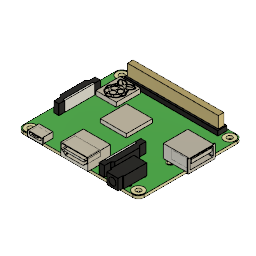
Raspberry PI 3 Model A+ - TG v7 (Autodesk Fusion 360 design; units mm, degrees)
Autodesk Fusion 360 part; units mm, degrees
note: some values were not read from the file. Set by a fixed rule: which sketch regions a step uses.
(part 1 of 2)
sketch "Board Outline" plane through (0, 0, 0) normal (0, 0, 1) x (1, 0, 0)
  arc A0 (0, 3) -> (3, 0) centre (3, 3) ccw
  line L0 (3, 0) -> (62, 0)
  line L1 (0, 53) -> (0, 3)
  arc A1 (3, 56) -> (0, 53) centre (3, 53) ccw
  circle A2 centre (61.5, 52.5) radius 3
  circle A3 centre (3.5, 52.5) radius 1.4
  arc A4 (65, 53) -> (62, 56) centre (62, 53) ccw
  circle A5 centre (61.5, 3.5) radius 1.4
  circle A6 centre (3.5, 3.5) radius 1.4
  arc A7 (62, 0) -> (65, 3) centre (62, 3) ccw
  circle A8 centre (61.5, 52.5) radius 1.4
  circle A9 centre (3.5, 52.5) radius 3
  circle A10 centre (61.5, 3.5) radius 3
  line L2 (65, 3) -> (65, 53)
  line L3 (62, 56) -> (3, 56)
  circle A11 centre (3.5, 3.5) radius 3
extrude "Extrude1" add sketch "Board Outline" along normal blind 1.5 contours A0 L0 L1 A1 A4 A7 L2 L3 makes body 1
extrude "Extrude2" add sketch "Board Outline" along normal blind 1.49 contours A2 | A9 | A10 | A11 bodies 1
sketch "Bottom Mounting Pads" plane through (0, 0, 0) normal (0, 0, -1) x (1, 0, 0)
  circle A0 centre (61.5, -3.5) radius 1.4
  circle A1 centre (3.5, -3.5) radius 1.4
  circle A2 centre (61.5, -52.5) radius 1.4
  circle A3 centre (3.5, -52.5) radius 1.4
  line L0 (3, -56) -> (62, -56)
  arc A4 (62, -56) -> (65, -53) centre (62, -53) ccw
  line L1 (65, -53) -> (65, -3)
  arc A5 (65, -3) -> (62, 0) centre (62, -3) ccw
  line L2 (62, 0) -> (3, 0)
  arc A6 (3, 0) -> (0, -3) centre (3, -3) ccw
  line L3 (0, -3) -> (0, -53)
  arc A7 (0, -53) -> (3, -56) centre (3, -53) ccw
extrude "Extrude3" cut sketch "Board Outline" along normal blind 0.01 contours A2 | A9 | A10 | A11 bodies 1
sketch "Components - Top" plane through (0, 0, 1.5) normal (0, 0, 1) x (1, 0, 0)
  line L0 (46.35, 19.35) -> (46.35, 22.7)
  line L1 (46.35, 22.7) -> (43.55, 22.7)
  line L2 (43.55, 22.7) -> (43.55, 0.3)
  line L3 (43.55, 3.5) -> (44.45, 3.5)
  line L4 (47.5, 4.8) -> (47.5, 18.2)
  line L5 (44.45, 19.5) -> (43.55, 19.5)
  line L6 (44.45, 3.5) -> (44.45, 19.5)
  line L7 (6.58, -1.22) -> (14.62, -1.22)
  line L8 (19.975, 24.525) -> (33.975, 24.525)
  line L9 (14.62, -1.22) -> (14.62, -0.6)
  line L10 (39.25, -1.5) -> (39.25, 10.65)
  line L11 (19.975, 38.525) -> (19.975, 24.525)
  line L12 (33.975, 38.525) -> (19.975, 38.525)
  line L13 (14.35, -0.6) -> (14.35, 4.71)
  line L14 (33.975, 24.525) -> (33.975, 38.525)
  line L15 (14.62, -0.6) -> (6.58, -0.6)
  line L16 (24.75, -1.5) -> (39.25, -1.5)
  line L17 (6.58, -0.6) -> (6.58, -1.22)
  line L18 (24.75, 10.65) -> (24.75, -1.5)
  line L19 (6.85, -0.6) -> (14.35, -0.6)
  line L20 (6.85, 4.71) -> (6.85, -0.6)
  line L21 (14.35, 4.71) -> (6.85, 4.71)
  line L22 (2.6, 39.2) -> (2.6, 35.8)
  line L23 (1.5, 21.3) -> (2.65, 20.15)
  line L24 (39.25, 10.65) -> (24.75, 10.65)
  line L25 (2.65, 20.15) -> (2.65, 16.8)
  line L26 (2.65, 16.8) -> (5.45, 16.8)
  line L27 (4.55, 20) -> (5.45, 20)
  line L28 (5.45, 16.8) -> (5.45, 39.2)
  line L29 (5.45, 36) -> (4.55, 36)
  line L30 (1.5, 34.7) -> (1.5, 21.3)
  line L31 (2.6, 35.8) -> (1.5, 34.7)
  line L32 (4.55, 36) -> (4.55, 20)
  line L33 (47.5, 18.2) -> (46.35, 19.35)
  line L34 (5.45, 39.2) -> (2.6, 39.2)
  line L35 (43.55, 0.3) -> (46.4, 0.3)
  line L36 (46.4, 0.3) -> (46.4, 3.7)
  line L37 (46.4, 3.7) -> (47.5, 4.8)
extrude "Extrude4" add sketch "Components - Top" along normal blind 2 separate body contours L8 L11 L12 L14 makes body 2
extrude "Extrude5" add sketch "Components - Top" along normal blind 5.5 separate body contours L0 L1 L2 L3 L4 L5 L6 L33 L35 L36 L37 | L22 L23 L25 L26 L27 L28 L29 L30 L31 L32 L34 makes body 3 at (4.55, 30.6667, 3.3333) makes body 4 at (44.45, 8.8333, 3.3333)
extrude "Extrude6" add sketch "Components - Top" along normal blind 5.51 separate body contours L2 L3 L5 L6 | L27 L28 L29 L32 makes body 5 at (5.45, 25.3333, 3.3367) makes body 6 at (44.45, 8.8333, 3.3367)
extrude "Extrude7" add sketch "Components - Top" along normal blind 6.5 separate body contours L10 L16 L18 L24 makes body 7
extrude "Extrude8" add sketch "Components - Top" along normal blind 3 separate body contours L7 L9 L15 L17 L19 | L13 L15 L19 L20 L21 makes body 8
sketch "Components - Bottom" plane through (0, 0, 0) normal (0, 0, -1) x (-1, 0, 0)
  line L0 (-13.135, 34.1) -> (-13.135, 22.11)
  line L1 (-1.685, 34.1) -> (-13.135, 34.1)
  line L2 (-13.135, 22.11) -> (-1.685, 22.11)
  line L3 (-1.685, 22.11) -> (-1.685, 34.1)
  line L4 (-1.685, 22.51) -> (2.265, 22.51)
  line L5 (-49.6, 39.5) -> (-37.6, 39.5)
  line L6 (2.265, 22.51) -> (2.265, 33.51)
  line L7 (2.265, 33.51) -> (-1.685, 33.51)
  line L8 (-37.6, 39.5) -> (-37.6, 27.5)
  line L9 (-37.6, 27.5) -> (-49.6, 27.5)
  line L10 (-49.6, 27.5) -> (-49.6, 39.5)
extrude "Extrude9" add sketch "Components - Bottom" along normal blind 0.65 separate body contours L5 L8 L9 L10 makes body 9
extrude "Extrude10" add sketch "Components - Bottom" along normal blind 1.45 separate body contours L0 L1 L2 L3 | L3 L4 L6 L7 makes body 10
sketch "Pads" plane through (0, 0, 1.5) normal (0, 0, 1) x (1, 0, 0)
  circle A0 centre (54.5, 30.45) radius 0.75
  circle A1 centre (56.63, 51.23) radius 0.8
  circle A2 centre (57.21, 24.88) radius 1.725
  circle A3 centre (8.37, 53.77) radius 0.8
  circle A4 centre (54.5, 27.95) radius 0.75
  circle A5 centre (50.3, 3.5) radius 0.9
  circle A6 centre (54.5, 32.45) radius 0.75
  circle A7 centre (54.5, 34.95) radius 0.75
  line L0 (9.17, 52.03) -> (9.17, 50.43)
  circle A8 centre (41.39, 51.23) radius 0.8
  circle A9 centre (41.39, 53.77) radius 0.8
  line L1 (7.57, 52.03) -> (9.17, 52.03)
  line L2 (7.57, 50.43) -> (7.57, 52.03)
  circle A10 centre (57.21, 38.02) radius 1.725
  line L3 (9.17, 50.43) -> (7.57, 50.43)
  circle A11 centre (46.47, 51.23) radius 0.8
  circle A12 centre (28.69, 53.77) radius 0.8
  circle A13 centre (38.85, 53.77) radius 0.8
  circle A14 centre (15.99, 51.23) radius 0.8
  circle A15 centre (54.09, 53.77) radius 0.8
  circle A16 centre (49.01, 51.23) radius 0.8
  circle A17 centre (13.45, 53.77) radius 0.8
  circle A18 centre (46.47, 53.77) radius 0.8
  circle A19 centre (21.07, 51.23) radius 0.8
  circle A20 centre (23.61, 51.23) radius 0.8
  circle A21 centre (36.31, 51.23) radius 0.8
  circle A22 centre (10.91, 53.77) radius 0.8
  circle A23 centre (43.93, 51.23) radius 0.8
  circle A24 centre (43.93, 53.77) radius 0.8
  circle A25 centre (21.07, 53.77) radius 0.8
  circle A26 centre (56.63, 53.77) radius 0.8
  circle A27 centre (13.45, 51.23) radius 0.8
  circle A28 centre (26.15, 53.77) radius 0.8
  circle A29 centre (50.6, 11.5) radius 0.475
  circle A30 centre (41.39, 53.77) radius 0.475
  circle A31 centre (36.31, 51.23) radius 0.475
  circle A32 centre (10.91, 51.23) radius 0.8
  circle A33 centre (23.61, 51.23) radius 0.475
  circle A34 centre (49.01, 53.77) radius 0.475
  circle A35 centre (49.01, 51.23) radius 0.475
  circle A36 centre (54.09, 51.23) radius 0.475
  circle A37 centre (28.69, 51.23) radius 0.8
  circle A38 centre (54.5, 34.95) radius 0.475
  circle A39 centre (43.93, 53.77) radius 0.475
  circle A40 centre (51.55, 51.23) radius 0.475
  circle A41 centre (23.61, 53.77) radius 0.8
  circle A42 centre (53.5, 12.2) radius 0.475
  circle A43 centre (56.63, 53.77) radius 0.475
  circle A44 centre (36.31, 53.77) radius 0.475
  circle A45 centre (46.47, 51.23) radius 0.475
  circle A46 centre (54.09, 53.77) radius 0.475
  circle A47 centre (38.85, 51.23) radius 0.475
  circle A48 centre (49.01, 53.77) radius 0.8
  circle A49 centre (54.5, 32.45) radius 0.475
  circle A50 centre (31.23, 53.77) radius 0.475
  circle A51 centre (18.53, 53.77) radius 0.8
  circle A52 centre (33.77, 51.23) radius 0.475
  circle A53 centre (15.99, 53.77) radius 0.8
  circle A54 centre (31.23, 51.23) radius 0.8
  circle A55 centre (54.09, 51.23) radius 0.8
  circle A56 centre (23.61, 53.77) radius 0.475
  circle A57 centre (50.3, 3.5) radius 0.475
  circle A58 centre (18.53, 51.23) radius 0.8
  circle A59 centre (31.23, 53.77) radius 0.8
  circle A60 centre (54.5, 27.95) radius 0.475
  circle A61 centre (53.5, 12.2) radius 0.9
  circle A62 centre (26.15, 53.77) radius 0.475
  circle A63 centre (51.55, 51.23) radius 0.8
  circle A64 centre (56.63, 51.23) radius 0.475
  circle A65 centre (46.47, 53.77) radius 0.475
  circle A66 centre (36.31, 53.77) radius 0.8
  circle A67 centre (33.77, 53.77) radius 0.8
  circle A68 centre (56.7, 3.5) radius 0.475
  circle A69 centre (56.7, 3.5) radius 0.9
  circle A70 centre (41.39, 51.23) radius 0.475
  circle A71 centre (57.21, 38.02) radius 1.15
  circle A72 centre (38.85, 53.77) radius 0.475
  circle A73 centre (57.21, 24.88) radius 1.15
  circle A74 centre (31.23, 51.23) radius 0.475
  circle A75 centre (56.4, 11.5) radius 0.475
  circle A76 centre (51.55, 53.77) radius 0.475
  circle A77 centre (38.85, 51.23) radius 0.8
  circle A78 centre (26.15, 51.23) radius 0.8
  circle A79 centre (43.93, 51.23) radius 0.475
  circle A80 centre (51.55, 53.77) radius 0.8
  circle A81 centre (33.77, 51.23) radius 0.8
  circle A82 centre (56.4, 11.5) radius 0.9
  circle A83 centre (54.5, 30.45) radius 0.475
  circle A84 centre (28.69, 53.77) radius 0.475
  circle A85 centre (50.6, 11.5) radius 0.9
  circle A86 centre (33.77, 53.77) radius 0.475
  circle A87 centre (8.37, 53.77) radius 0.475
  circle A88 centre (15.99, 53.77) radius 0.475
  circle A89 centre (13.45, 51.23) radius 0.475
  circle A90 centre (10.91, 53.77) radius 0.475
  circle A91 centre (10.91, 51.23) radius 0.475
  circle A92 centre (15.99, 51.23) radius 0.475
  circle A93 centre (21.07, 53.77) radius 0.475
  circle A94 centre (28.69, 51.23) radius 0.475
  circle A95 centre (21.07, 51.23) radius 0.475
  circle A96 centre (8.37, 51.23) radius 0.475
  circle A97 centre (13.45, 53.77) radius 0.475
  circle A98 centre (18.53, 53.77) radius 0.475
  circle A99 centre (18.53, 51.23) radius 0.475
  circle A100 centre (26.15, 51.23) radius 0.475
extrude "Extrude11" cut sketch "Pads" against normal blind 0.01 contours L0 L1 L2 L3 bodies 1
hole "Hole2" at (56.63, 53.77, 1.5) direction (0, 0, -1) diameter 0.95 depth 1.5 tip angle 118 counterbore diameter 1.6 counterbore depth 0.01 bodies 1
sketch "Sketch14" plane through (0, 0, 0) normal (0, 0, -1) x (1, 0, 0)
  line L0 (3, -56) -> (62, -56)
  arc A0 (62, -56) -> (65, -53) centre (62, -53) ccw
  line L1 (65, -53) -> (65, -3)
  arc A1 (65, -3) -> (62, 0) centre (62, -3) ccw
  line L2 (62, 0) -> (3, 0)
  arc A2 (3, 0) -> (0, -3) centre (3, -3) ccw
  line L3 (0, -3) -> (0, -53)
  arc A3 (0, -53) -> (3, -56) centre (3, -53) ccw
  circle A4 centre (56.63, -53.77) radius 0.8
  circle A5 centre (61.5, -3.5) radius 3
  circle A6 centre (61.5, -52.5) radius 3
  circle A7 centre (3.5, -3.5) radius 3
  circle A8 centre (3.5, -52.5) radius 3
  circle A9 centre (56.63, -53.77) radius 0.475
extrude "Extrude12" cut sketch "Sketch14" against normal blind 0.01 contours A4 bodies 1
pattern_linear "R-Pattern1" count 20 spacing 2.54 along (-1, 0, 0) count 2 spacing 2.54 along (0, -1, 0) of "Hole2", "Extrude12"
extrude "Extrude13" cut sketch "Pads" against normal up to surface (1.5 mm away) contours A29 | A38 | A42 | A49 | A57 | A60 | A68 | A71 | A73 | A75 | A83 bodies 1
extrude "Extrude14" cut sketch "Pads" against normal blind 0.01 contours A0 | A2 | A4 | A5 | A6 | A7 | A10 | A61 | A69 | A82 | A85 bodies 1
sketch "Additional Components" plane through (0, 0, 1.5) normal (0, 0, 1) x (1, 0, 0)
  line L0 (8.425, 1.95) -> (8.425, 1.25)
  line L1 (7.325, 1.25) -> (7.325, 1.95)
  line L2 (50, 12.5) -> (50, 0)
  line L3 (56.5, -2.5) -> (56.5, 0)
  arc A0 (12.775, 1.95) -> (13.875, 1.95) centre (13.325, 1.95) cw
  line L4 (56.5, 0) -> (50.5, 0)
  line L5 (50.5, 0) -> (50.5, -2.5)
  arc A1 (8.7, 4.43) -> (7.65, 4.43) centre (8.175, 4.43) cw
  line L6 (67.5, 38.02) -> (67.5, 38.8)
  line L7 (12.5, 4.43) -> (12.5, 4.83)
  line L8 (13.55, 4.83) -> (13.55, 4.43)
  line L9 (13.875, 1.95) -> (13.875, 1.25)
  arc A2 (7.325, 1.95) -> (8.425, 1.95) centre (7.875, 1.95) cw
  line L10 (67.5, 38.8) -> (67, 38.8)
  line L11 (12.775, 1.25) -> (12.775, 1.95)
  arc A3 (13.875, 1.25) -> (12.775, 1.25) centre (13.325, 1.25) cw
  arc A4 (12.5, 4.83) -> (13.55, 4.83) centre (13.025, 4.83) cw
  line L12 (8.7, 4.83) -> (8.7, 4.43)
  line L13 (53.5, 24.88) -> (53.5, 38.02)
  line L14 (67, 24.1) -> (67, 24.88)
  line L15 (67.5, 24.88) -> (53.5, 24.88)
  line L16 (67.5, 38.02) -> (67.5, 24.1)
  line L17 (7.65, 4.43) -> (7.65, 4.83)
  arc A5 (7.65, 4.83) -> (8.7, 4.83) centre (8.175, 4.83) cw
  line L18 (67, 38.8) -> (67, 38.02)
  line L19 (57, 0) -> (57, 12.5)
  arc A6 (13.55, 4.43) -> (12.5, 4.43) centre (13.025, 4.43) cw
  arc A7 (8.425, 1.25) -> (7.325, 1.25) centre (7.875, 1.25) cw
  line L20 (67.5, 24.1) -> (67, 24.1)
  line L21 (57, 12.5) -> (50, 12.5)
  arc A8 (8.5, 4.43) -> (7.85, 4.43) centre (8.175, 4.43) cw
  line L22 (7.525, 1.25) -> (7.525, 1.95)
  line L23 (50, 0) -> (57, 0)
  arc A9 (24, 3.49) -> (25.5, 3.49) centre (24.75, 3.49) cw
  arc A10 (38.5, 9.95) -> (40, 9.95) centre (39.25, 9.95) cw
  arc A11 (7.85, 4.83) -> (8.5, 4.83) centre (8.175, 4.83) cw
  line L24 (12.7, 4.43) -> (12.7, 4.83)
  line L25 (53.5, 38.02) -> (67.5, 38.02)
  arc A12 (38.5, 3.49) -> (40, 3.49) centre (39.25, 3.49) cw
  arc A13 (40, 8.15) -> (38.5, 8.15) centre (39.25, 8.15) cw
  line L26 (24, 8.15) -> (24, 9.95)
  arc A14 (25.5, 8.15) -> (24, 8.15) centre (24.75, 8.15) cw
  arc A15 (8.5, 4.43) -> (7.85, 4.43) centre (8.175, 4.43) cw
  line L27 (8.5, 4.83) -> (8.5, 4.43)
  line L28 (7.85, 4.43) -> (7.85, 4.83)
  line L29 (25.5, 9.95) -> (25.5, 8.15)
  arc A16 (13.35, 4.43) -> (12.7, 4.43) centre (13.025, 4.43) cw
  arc A17 (8.225, 1.25) -> (7.525, 1.25) centre (7.875, 1.25) cw
  line L30 (13.35, 4.83) -> (13.35, 4.43)
  line L31 (40, 3.49) -> (40, 2.69)
  line L32 (24, 2.69) -> (24, 3.49)
  line L33 (25.5, 3.49) -> (25.5, 2.69)
  line L34 (40, 9.95) -> (40, 8.15)
  line L35 (7.85, 4.43) -> (7.85, 4.83)
  line L36 (7.85, 4.43) -> (7.85, 4.83)
  arc A18 (7.85, 4.83) -> (8.5, 4.83) centre (8.175, 4.83) cw
  arc A19 (7.85, 4.83) -> (8.5, 4.83) centre (8.175, 4.83) cw
  arc A20 (40, 2.69) -> (38.5, 2.69) centre (39.25, 2.69) cw
  arc A21 (24, 9.95) -> (25.5, 9.95) centre (24.75, 9.95) cw
  arc A22 (7.525, 1.95) -> (8.225, 1.95) centre (7.875, 1.95) cw
  line L37 (50.5, -2.5) -> (56.5, -2.5)
  line L38 (38.5, 2.69) -> (38.5, 3.49)
  line L39 (38.5, 8.15) -> (38.5, 9.95)
  line L40 (8.5, 4.83) -> (8.5, 4.43)
  line L41 (8.225, 1.95) -> (8.225, 1.25)
  arc A23 (7.85, 4.83) -> (8.5, 4.83) centre (8.175, 4.83) cw
  line L42 (8.5, 4.83) -> (8.5, 4.43)
  line L43 (8.5, 4.83) -> (8.5, 4.43)
  arc A24 (25.5, 2.69) -> (24, 2.69) centre (24.75, 2.69) cw
  arc A25 (12.975, 1.95) -> (13.675, 1.95) centre (13.325, 1.95) cw
  arc A26 (8.5, 4.43) -> (7.85, 4.43) centre (8.175, 4.43) cw
  arc A27 (39.8, 2.69) -> (38.7, 2.69) centre (39.25, 2.69) cw
  line L44 (38.7, 8.15) -> (38.7, 9.95)
  line L45 (8.5, 4.83) -> (8.5, 4.43)
  line L46 (12.975, 1.25) -> (12.975, 1.95)
  arc A28 (8.5, 4.43) -> (7.85, 4.43) centre (8.175, 4.43) cw
  line L47 (38.7, 2.69) -> (38.7, 3.49)
  line L48 (25.3, 3.49) -> (25.3, 2.69)
  line L49 (25.3, 9.95) -> (25.3, 8.15)
  arc A29 (12.7, 4.83) -> (13.35, 4.83) centre (13.025, 4.83) cw
  arc A30 (24.2, 9.95) -> (25.3, 9.95) centre (24.75, 9.95) cw
  arc A31 (8.5, 4.43) -> (7.85, 4.43) centre (8.175, 4.43) cw
  arc A32 (38.7, 9.95) -> (39.8, 9.95) centre (39.25, 9.95) cw
  arc A33 (8.5, 4.43) -> (7.85, 4.43) centre (8.175, 4.43) cw
  line L50 (39.8, 9.95) -> (39.8, 8.15)
  arc A34 (13.675, 1.25) -> (12.975, 1.25) centre (13.325, 1.25) cw
  line L51 (24.2, 2.69) -> (24.2, 3.49)
  line L52 (24.2, 8.15) -> (24.2, 9.95)
  line L53 (13.675, 1.95) -> (13.675, 1.25)
  line L54 (39.8, 3.49) -> (39.8, 2.69)
  arc A35 (25.3, 8.15) -> (24.2, 8.15) centre (24.75, 8.15) cw
  line L55 (7.85, 4.43) -> (7.85, 4.83)
  line L56 (8.5, 4.83) -> (8.5, 4.43)
  line L57 (7.85, 4.43) -> (7.85, 4.83)
  arc A36 (7.85, 4.83) -> (8.5, 4.83) centre (8.175, 4.83) cw
  line L58 (7.85, 4.43) -> (7.85, 4.83)
  arc A37 (38.7, 3.49) -> (39.8, 3.49) centre (39.25, 3.49) cw
  arc A38 (25.3, 2.69) -> (24.2, 2.69) centre (24.75, 2.69) cw
  arc A39 (7.85, 4.83) -> (8.5, 4.83) centre (8.175, 4.83) cw
  arc A40 (39.8, 8.15) -> (38.7, 8.15) centre (39.25, 8.15) cw
  arc A41 (8.5, 4.43) -> (7.85, 4.43) centre (8.175, 4.43) cw
  arc A42 (7.85, 4.83) -> (8.5, 4.83) centre (8.175, 4.83) cw
  line L59 (8.5, 4.83) -> (8.5, 4.43)
  arc A43 (7.85, 4.83) -> (8.5, 4.83) centre (8.175, 4.83) cw
  line L60 (7.85, 4.43) -> (7.85, 4.83)
  line L61 (7.85, 4.43) -> (7.85, 4.83)
  arc A44 (8.5, 4.43) -> (7.85, 4.43) centre (8.175, 4.43) cw
  arc A45 (24.2, 3.49) -> (25.3, 3.49) centre (24.75, 3.49) cw
  line L62 (8.5, 4.83) -> (8.5, 4.43)
  line L63 (6, 49.1) -> (17, 49.1)
  line L64 (17, 49.1) -> (17, 36.1)
  line L65 (17, 36.1) -> (6, 36.1)
  line L66 (6, 36.1) -> (6, 49.1)
  line L67 (62, 56) -> (3, 56)
  line L68 (0, 53) -> (0, 3)
  line L69 (57.625, 55) -> (7.375, 55)
  line L70 (7.375, 55) -> (7.375, 50)
  line L71 (7.375, 50) -> (57.625, 50)
  line L72 (57.625, 50) -> (57.625, 55)
  line L73 (57.625, 55) -> (7.375, 50) construction
  line L74 (7.375, 55) -> (57.625, 50) construction
  dimension "d51" = 11
  dimension "d52" = 13
  dimension "d53" = 19.9
  dimension "d54" = 17
  dimension "d57" = 50.25
  dimension "d58" = 5
  dimension "d59" = 32.5
  dimension "d60" = 3.5
  measures "d53" distance of L65 L67
  measures "d54" distance of L64 L68
  measures "d57" distance of origin
  measures "d60" distance of L67 origin
extrude "Extrude19" add sketch "Additional Components" along normal blind 2.5 separate body contours L69 L70 L71 L72 makes body 11
extrude "Extrude15" add sketch "Additional Components" along normal blind 6 separate body contours L2 L4 L19 L21 L23 | L3 L4 L5 L23 L37 makes body 12
sketch "Sketch17" plane through (0, -2.5, 0) normal (0, -1, 0) x (1, 0, 0)
  line L0 (50.5, 1.5) -> (56.5, 1.5)
  line L1 (56.5, 1.5) -> (56.5, 7.5)
  line L2 (56.5, 7.5) -> (50.5, 7.5)
  line L3 (50.5, 7.5) -> (50.5, 1.5)
  line L4 (50.5, 7.5) -> (56.5, 1.5) construction
  line L5 (56.5, 7.5) -> (50.5, 1.5) construction
  circle A0 centre (53.5, 4.5) radius 1.875
  dimension "d46" = 3.75
  measures "d46" diameter of A0
extrude "Extrude16" cut sketch "Sketch17" against normal blind 10 contours A0 bodies 12
extrude "Extrude17" add sketch "Additional Components" along normal blind 7.1 separate body contours L6 L10 L18 L25 | L13 L15 L16 L25 | L14 L15 L16 L20 makes body 13
extrude "Extrude18" add sketch "Additional Components" along normal blind 2.35 separate body contours L63 L64 L65 L66 makes body 14
sketch "Sketch18" plane through (0, 0, 4) normal (0, 0, 1) x (-1, 0, 0)
  line L0 (-57.625, -50) -> (-57.625, -55)
  line L1 (-57.625, -55) -> (-7.375, -55)
  line L2 (-7.375, -55) -> (-7.375, -50)
  line L3 (-7.375, -50) -> (-57.625, -50)
  line L4 (-56.95, -50.95) -> (-8.05, -50.95)
  line L5 (-8.05, -50.95) -> (-8.05, -54.05)
  line L6 (-8.05, -54.05) -> (-56.95, -54.05)
  line L7 (-56.95, -54.05) -> (-56.95, -50.95)
  line L8 (-56.95, -50.95) -> (-8.05, -54.05) construction
  line L9 (-8.05, -50.95) -> (-56.95, -54.05) construction
  dimension "d63" = 48.9
  dimension "d64" = 3.1
  measures "d63" distance of origin
extrude "Extrude20" add sketch "Sketch18" along normal blind 6.2 separate body contours L4 L5 L6 L7 makes body 15
sketch "USB" plane through (67.5, 0, 0) normal (1, 0, 0) x (0, 1, 0)
  line L0 (25.9, 7.53) -> (25.9, 5.69)
  line L1 (25.203, 7.79) -> (25.203, 3.31)
  arc A0 (25.523, 8.11) -> (25.203, 7.79) centre (25.523, 7.79) ccw
  line L2 (37.377, 8.11) -> (25.523, 8.11)
  line L3 (25.203, 3.31) -> (25.203, 3.31)
  line L4 (37, 7.53) -> (25.9, 7.53)
  line L5 (37, 5.69) -> (37, 7.53)
  arc A1 (37.377, 2.99) -> (37.697, 3.31) centre (37.377, 3.31) ccw
  line L6 (25.203, 3.31) -> (25.203, 3.31)
  line L7 (37.697, 7.79) -> (37.697, 7.79)
  line L8 (37.697, 3.31) -> (37.697, 7.79)
  line L9 (25.523, 2.99) -> (37.377, 2.99)
  arc A2 (25.203, 3.31) -> (25.523, 2.99) centre (25.523, 3.31) ccw
  line L10 (37.377, 2.99) -> (37.377, 2.99)
  line L11 (37.697, 7.79) -> (37.697, 7.79)
  line L12 (37.377, 2.99) -> (37.377, 2.99)
  line L13 (25.9, 5.69) -> (37, 5.69)
  arc A3 (37.697, 7.79) -> (37.377, 8.11) centre (37.377, 7.79) ccw
extrude "Extrude21" cut sketch "USB" against normal blind 10 bodies 13
sketch "HDMI (1)" plane through (32, -1.5, 5.4) normal (0, -1, 0) x (1, 0, 0)
  arc A0 (-5.2, 0.5825) -> (-5.6, 0.1825) centre (-5.2, 0.1825) ccw
  line L0 (-5.6852, -1.3589) -> (-5.1001, -2.0879)
  arc A1 (7, 1.775) -> (6.5, 2.275) centre (6.5, 1.775) ccw
  line L1 (5.1001, -2.0879) -> (5.6852, -1.3589)
  arc A2 (4.7, -0.5825) -> (4.8143, -0.5658) centre (4.7, -0.1825) ccw
  arc A3 (-5.1001, -2.0879) -> (-4.7102, -2.275) centre (-4.7102, -1.775) ccw
  arc A4 (-6.5, 2.275) -> (-7, 1.775) centre (-6.5, 1.775) ccw
  line L2 (6.5, 2.275) -> (-6.5, 2.275)
  arc A5 (5.6852, -1.3589) -> (6.7075, -0.775) centre (7.4252, -3.2186) cw
  line L3 (5.6, -0.0334) -> (5.6, 0.1825)
  arc A6 (-7, -0.3201) -> (-6.7075, -0.775) centre (-6.5, -0.3201) ccw
  arc A7 (5.6, 0.1825) -> (5.2, 0.5825) centre (5.2, 0.1825) ccw
  line L4 (-7, 1.775) -> (-7, -0.3201)
  line L5 (5.2, 0.5825) -> (-5.2, 0.5825)
  line L6 (4.8143, -0.5658) -> (5.3143, -0.4168)
  line L7 (-4.7102, -2.275) -> (4.7102, -2.275)
  arc A8 (5.3143, -0.4168) -> (5.6, -0.0334) centre (5.2, -0.0334) ccw
  arc A9 (6.7075, -0.775) -> (7, -0.3201) centre (6.5, -0.3201) ccw
  line L8 (-5.6, 0.1825) -> (-5.6, -0.0334)
  line L9 (-6.7075, -0.775) -> (-6.05, -1.075)
  arc A10 (-6.05, -1.075) -> (-5.6852, -1.3589) centre (-6.4651, -1.9848) cw
  arc A11 (-5.6, -0.0334) -> (-5.3143, -0.4168) centre (-5.2, -0.0334) ccw
  arc A12 (4.7102, -2.275) -> (5.1001, -2.0879) centre (4.7102, -1.775) ccw
  line L10 (7, -0.3201) -> (7, 1.775)
  line L11 (-5.3143, -0.4168) -> (-4.8143, -0.5658)
  arc A13 (-4.8143, -0.5658) -> (-4.7, -0.5825) centre (-4.7, -0.1825) ccw
  line L12 (-4.7, -0.5825) -> (4.7, -0.5825)
extrude "Extrude22" cut sketch "HDMI (1)" against normal blind 7 bodies 7
sketch "MicroUSB" plane through (10.7, -1.22, 3.4) normal (0, -1, 0) x (1, 0, 0)
  arc A0 (1.5, -0.025) -> (1.7, 0.175) centre (1.5, 0.175) ccw
  line L0 (1.7, 0.175) -> (1.7, 0.375)
  line L1 (-3.24, 0.665) -> (-3.24, -0.0673)
  arc A1 (-3.24, -0.0673) -> (-3.2254, -0.1027) centre (-3.19, -0.0673) ccw
  arc A2 (-1.5, 0.575) -> (-1.7, 0.375) centre (-1.5, 0.375) ccw
  arc A3 (3.24, 0.665) -> (3.19, 0.715) centre (3.19, 0.665) ccw
  line L2 (3.24, -0.0673) -> (3.24, 0.665)
  line L3 (1.5, 0.575) -> (-1.5, 0.575)
  arc A4 (-3.19, 0.715) -> (-3.24, 0.665) centre (-3.19, 0.665) ccw
  line L4 (-1.5, -0.025) -> (1.5, -0.025)
  line L5 (-1.7, 0.375) -> (-1.7, 0.175)
  line L6 (3.19, 0.715) -> (-3.19, 0.715)
  arc A5 (-1.7, 0.175) -> (-1.5, -0.025) centre (-1.5, 0.175) ccw
  arc A6 (1.7, 0.375) -> (1.5, 0.575) centre (1.5, 0.375) ccw
  line L7 (-3.2254, -0.1027) -> (-2.5923, -0.715)
  line L8 (2.5923, -0.715) -> (3.2254, -0.1027)
  arc A7 (3.2254, -0.1027) -> (3.24, -0.0673) centre (3.19, -0.0673) ccw
  line L9 (-2.5923, -0.715) -> (2.5923, -0.715)
extrude "Extrude23" cut sketch "MicroUSB" against normal blind 4.6 bodies 8
sketch "rpi3" plane through (6, 36, 3.85) normal (0, 0, 1) x (1, 0, 0)
  spline S0 degree 3 poles (8.4596, 11.9282) (8.4178, 11.9443) (8.4164, 12.0305) (8.4574, 12.0645) knots 0 0 0 0 1 1 1 1
  spline S1 degree 3 poles (8.2654, 12.0534) (7.9941, 11.9818) (7.9366, 12.0064) (8.0525, 12.1442) knots 0 0 0 0 1 1 1 1
  spline S2 degree 3 poles (7.5949, 12.1687) (7.612, 12.2007) (7.591, 12.1933) (7.4984, 12.1347) knots 0 0 0 0 1 1 1 1
  spline S3 degree 3 poles (7.8457, 9.257) (7.8745, 9.2439) (7.8981, 9.2219) (7.8981, 9.2081) knots 0 0 0 0 1 1 1 1
  spline S4 degree 3 poles (7.4984, 12.1347) (7.4332, 12.0935) (7.3566, 12.0379) (7.328, 12.0112) knots 0 0 0 0 1 1 1 1
  line L0 (9.0436, 11.9829) -> (8.9839, 11.9857)
  line L1 (8.7312, 9.9095) -> (8.5991, 9.8422)
  line L2 (8.989, 11.9259) -> (9.0436, 11.9829)
  spline S5 degree 3 poles (7.7199, 12.0493) (7.6496, 12.0084) (7.6274, 12.0036) (7.603, 12.0238) knots 0 0 0 0 1 1 1 1
  spline S6 degree 3 poles (7.956, 12.1534) (7.8739, 12.1239) (7.7676, 12.0771) (7.7199, 12.0493) knots 0 0 0 0 1 1 1 1
  spline S7 degree 3 poles (8.6272, 11.9486) (8.5533, 11.9304) (8.4778, 11.9212) (8.4596, 11.9282) knots 0 0 0 0 1 1 1 1
  spline S8 degree 3 poles (8.4574, 12.0645) (8.513, 12.1107) (8.4741, 12.1084) (8.2654, 12.0534) knots 0 0 0 0 1 1 1 1
  spline S9 degree 3 poles (7.603, 12.0238) (7.5676, 12.0533) (7.5643, 12.1116) (7.5949, 12.1687) knots 0 0 0 0 1 1 1 1
  spline S10 degree 3 poles (7.8981, 9.2081) (7.8981, 9.1555) (7.8128, 9.1495) (7.4991, 9.1799) knots 0 0 0 0 1 1 1 1
  spline S11 degree 3 poles (7.7691, 9.2565) (7.7254, 9.3049) (7.7263, 9.3563) (7.7711, 9.3687) knots 0 0 0 0 1 1 1 1
  spline S12 degree 3 poles (8.2544, 9.4866) (8.2261, 9.5089) (8.2029, 9.5394) (8.2029, 9.5544) knots 0 0 0 0 1 1 1 1
  spline S13 degree 3 poles (7.7711, 9.3687) (7.7906, 9.3742) (7.8706, 9.3843) (7.9489, 9.3913) knots 0 0 0 0 1 1 1 1
  spline S14 degree 3 poles (7.9489, 9.3913) (8.0271, 9.3983) (8.1394, 9.4135) (8.1985, 9.425) knots 0 0 0 0 1 1 1 1
  spline S15 degree 3 poles (8.4213, 9.6549) (8.7026, 9.749) (8.7145, 9.7569) (8.6219, 9.7875) knots 0 0 0 0 1 1 1 1
  line L3 (8.5991, 9.8422) -> (8.6866, 9.8203)
  spline S16 degree 3 poles (4.6931, 11.8745) (4.7268, 11.8954) (4.93, 11.6608) (5.0437, 11.4696) knots 0 0 0 0 1 1 1 1
  spline S17 degree 3 poles (5.0437, 11.4696) (5.2567, 11.1116) (5.3236, 10.7444) (5.2187, 10.5097) knots 0 0 0 0 1 1 1 1
  spline S18 degree 3 poles (4.657, 11.7997) (4.6643, 11.8331) (4.6806, 11.8668) (4.6931, 11.8745) knots 0 0 0 0 1 1 1 1
  spline S19 degree 3 poles (8.8584, 10.2168) (8.8557, 10.2326) (8.9086, 10.2821) (8.9759, 10.3268) knots 0 0 0 0 1 1 1 1
  spline S20 degree 3 poles (5.2187, 10.5097) (5.1643, 10.3879) (5.017, 10.2323) (4.9108, 10.1844) knots 0 0 0 0 1 1 1 1
  spline S21 degree 3 poles (3.3921, 12.0642) (3.4182, 12.0641) (3.4089, 12.1191) (3.3722, 12.1831) knots 0 0 0 0 1 1 1 1
  spline S22 degree 3 poles (3.5902, 10.9469) (3.3766, 11.0543) (2.9158, 11.2542) (2.9056, 11.244) knots 0 0 0 0 1 1 1 1
  line L4 (9.3588, 10.9101) -> (9.4073, 10.9652)
  line L5 (9.1626, 10.4741) -> (9.2269, 10.5401)
  line L6 (9.0224, 10.1436) -> (8.9428, 10.1659)
  spline S23 degree 3 poles (8.2029, 9.5544) (8.2029, 9.5711) (8.2882, 9.6103) (8.4213, 9.6549) knots 0 0 0 0 1 1 1 1
  spline S24 degree 3 poles (3.3517, 12.259) (3.3747, 12.2821) (3.5275, 12.2053) (3.6653, 12.1014) knots 0 0 0 0 1 1 1 1
  spline S25 degree 3 poles (9.4043, 11.7222) (9.4277, 11.7551) (9.4405, 11.7883) (9.4328, 11.7961) knots 0 0 0 0 1 1 1 1
  spline S26 degree 3 poles (4.6355, 11.739) (4.64, 11.739) (4.6497, 11.7663) (4.657, 11.7997) knots 0 0 0 0 1 1 1 1
  line L7 (9.4073, 10.9652) -> (9.3362, 10.9537)
  spline S27 degree 3 poles (8.7058, 9.9522) (8.7924, 9.9997) (8.8991, 10.0622) (8.9428, 10.0911) knots 0 0 0 0 1 1 1 1
  spline S28 degree 3 poles (9.0856, 10.571) (9.0477, 10.6006) (9.0515, 10.6069) (9.1782, 10.7285) knots 0 0 0 0 1 1 1 1
  line L8 (2.0332, 11.8609) -> (1.9747, 11.922)
  spline S29 degree 3 poles (2.9056, 11.244) (2.9014, 11.2399) (3.0204, 11.1669) (3.1699, 11.0819) knots 0 0 0 0 1 1 1 1
  spline S30 degree 3 poles (3.1699, 11.0819) (3.718, 10.7703) (4.3245, 10.3345) (4.5847, 10.0653) knots 0 0 0 0 1 1 1 1
  line L9 (4.9108, 10.1844) -> (4.8338, 10.1497)
  spline S31 degree 3 poles (9.1759, 10.5401) (9.148, 10.5401) (9.1073, 10.554) (9.0856, 10.571) knots 0 0 0 0 1 1 1 1
  line L10 (1.7754, 11.8609) -> (2.0332, 11.8609)
  spline S32 degree 3 poles (4.6337, 10.3017) (4.3246, 10.5365) (3.9674, 10.7573) (3.5902, 10.9469) knots 0 0 0 0 1 1 1 1
  spline S33 degree 3 poles (3.8229, 12.1337) (3.8132, 12.185) (3.8166, 12.2064) (3.8342, 12.2064) knots 0 0 0 0 1 1 1 1
  line L11 (4.8338, 10.1497) -> (4.6337, 10.3017)
  line L12 (4.5847, 10.0653) -> (4.6749, 9.972)
  spline S34 degree 3 poles (4.6399, 9.861) (4.5525, 9.5838) (4.2856, 9.36) (3.9148, 9.253) knots 0 0 0 0 1 1 1 1
  line L13 (9.2269, 10.5401) -> (9.1759, 10.5401)
  line L14 (8.1985, 9.425) -> (8.3059, 9.446)
  spline S35 degree 3 poles (9.1782, 10.7285) (9.2509, 10.7981) (9.3321, 10.8799) (9.3588, 10.9101) knots 0 0 0 0 1 1 1 1
  spline S36 degree 3 poles (8.5483, 9.8388) (8.5483, 9.8537) (8.6192, 9.9047) (8.7058, 9.9522) knots 0 0 0 0 1 1 1 1
  spline S37 degree 3 poles (9.1782, 11.0118) (9.1782, 11.0246) (9.2491, 11.1089) (9.3357, 11.1991) knots 0 0 0 0 1 1 1 1
  spline S38 degree 3 poles (9.1765, 11.8174) (9.0198, 11.822) (8.9344, 11.8324) (8.9344, 11.8467) knots 0 0 0 0 1 1 1 1
  spline S39 degree 3 poles (8.6219, 9.7875) (8.5814, 9.8008) (8.5483, 9.824) (8.5483, 9.8388) knots 0 0 0 0 1 1 1 1
  spline S40 degree 3 poles (8.9839, 11.9857) (8.8614, 11.9915) (8.7579, 11.9808) (8.6272, 11.9486) knots 0 0 0 0 1 1 1 1
  line L15 (9.4932, 11.3631) -> (9.3865, 11.3692)
  spline S41 degree 3 poles (8.9344, 11.8467) (8.9344, 11.8589) (8.959, 11.8945) (8.989, 11.9259) knots 0 0 0 0 1 1 1 1
  spline S42 degree 3 poles (3.3722, 12.1831) (3.3528, 12.2168) (3.3436, 12.251) (3.3517, 12.259) knots 0 0 0 0 1 1 1 1
  line L16 (8.9428, 10.0911) -> (9.0224, 10.1436)
  spline S43 degree 3 poles (3.6653, 12.1014) (3.8079, 11.9939) (3.8476, 12.0021) (3.8229, 12.1337) knots 0 0 0 0 1 1 1 1
  spline S44 degree 3 poles (4.1167, 11.9954) (4.1548, 11.9559) (4.1937, 11.9282) (4.2031, 11.934) knots 0 0 0 0 1 1 1 1
  spline S45 degree 3 poles (4.2031, 11.934) (4.2125, 11.9399) (4.2202, 11.9807) (4.2202, 12.0247) knots 0 0 0 0 1 1 1 1
  spline S46 degree 3 poles (8.9759, 10.3268) (9.0432, 10.3715) (9.1272, 10.4378) (9.1626, 10.4741) knots 0 0 0 0 1 1 1 1
  line L17 (9.3357, 11.1991) -> (9.4932, 11.3631)
  spline S47 degree 3 poles (9.3362, 10.9537) (9.2616, 10.9416) (9.1782, 10.9723) (9.1782, 11.0118) knots 0 0 0 0 1 1 1 1
  spline S48 degree 3 poles (4.5411, 11.8355) (4.5885, 11.7825) (4.6311, 11.739) (4.6355, 11.739) knots 0 0 0 0 1 1 1 1
  line L18 (8.3059, 9.446) -> (8.2544, 9.4866)
  spline S49 degree 3 poles (9.2798, 11.4234) (9.2798, 11.4816) (9.3459, 11.6402) (9.4043, 11.7222) knots 0 0 0 0 1 1 1 1
  spline S50 degree 3 poles (9.3865, 11.3692) (9.2896, 11.3748) (9.2798, 11.3798) (9.2798, 11.4234) knots 0 0 0 0 1 1 1 1
  spline S51 degree 3 poles (9.4328, 11.7961) (9.425, 11.8038) (9.3097, 11.8134) (9.1765, 11.8174) knots 0 0 0 0 1 1 1 1
  spline S52 degree 3 poles (3.8342, 12.2064) (3.8677, 12.2064) (4.031, 12.0844) (4.1167, 11.9954) knots 0 0 0 0 1 1 1 1
  spline S53 degree 3 poles (8.9428, 10.1659) (8.8991, 10.1781) (8.8611, 10.2011) (8.8584, 10.2168) knots 0 0 0 0 1 1 1 1
  spline S54 degree 3 poles (3.3092, 12.1055) (3.3464, 12.0829) (3.3837, 12.0643) (3.3921, 12.0642) knots 0 0 0 0 1 1 1 1
  spline S55 degree 3 poles (4.2202, 12.0247) (4.2202, 12.0819) (4.2288, 12.1048) (4.2503, 12.1048) knots 0 0 0 0 1 1 1 1
  spline S56 degree 3 poles (4.2503, 12.1048) (4.2814, 12.1048) (4.3909, 12.0034) (4.5411, 11.8355) knots 0 0 0 0 1 1 1 1
  line L19 (1.7946, 10.5292) -> (1.9254, 10.426)
  spline S57 degree 3 poles (2.3151, 9.9595) (2.4145, 9.9082) (2.4918, 9.8558) (2.4876, 9.8426) knots 0 0 0 0 1 1 1 1
  spline S58 degree 3 poles (1.863, 11.0071) (1.863, 10.9749) (1.758, 10.9423) (1.6949, 10.9548) knots 0 0 0 0 1 1 1 1
  spline S59 degree 3 poles (2.0671, 10.1026) (2.1044, 10.0751) (2.216, 10.0107) (2.3151, 9.9595) knots 0 0 0 0 1 1 1 1
  line L20 (4.6749, 9.972) -> (4.6399, 9.861)
  spline S60 degree 3 poles (4.6096, 10.3826) (4.7862, 10.251) (4.8482, 10.2152) (4.8839, 10.2242) knots 0 0 0 0 1 1 1 1
  spline S61 degree 3 poles (3.4226, 12.1843) (3.4559, 12.1493) (3.4551, 12.0547) (3.4213, 12.0266) knots 0 0 0 0 1 1 1 1
  line L21 (2.0836, 10.1661) -> (1.9993, 10.1526)
  line L22 (1.6436, 11.8079) -> (1.5817, 11.7955)
  spline S62 degree 3 poles (4.2608, 11.9739) (4.243, 11.8363) (4.1978, 11.8354) (4.0645, 11.9698) knots 0 0 0 0 1 1 1 1
  line L23 (1.5278, 11.3631) -> (1.6954, 11.1955)
  line L24 (4.8289, 11.6893) -> (4.7213, 11.8245)
  line L25 (2.413, 9.7867) -> (2.3461, 9.7546)
  spline S63 degree 3 poles (2.445, 9.713) (2.4993, 9.6901) (2.6055, 9.6512) (2.6809, 9.6266) knots 0 0 0 0 1 1 1 1
  spline S64 degree 3 poles (2.7404, 11.3659) (3.4039, 11.1256) (4.1131, 10.7525) (4.6096, 10.3826) knots 0 0 0 0 1 1 1 1
  spline S65 degree 3 poles (1.821, 10.754) (1.9, 10.6761) (1.9646, 10.6012) (1.9646, 10.5876) knots 0 0 0 0 1 1 1 1
  spline S66 degree 3 poles (2.7741, 9.4401) (2.7993, 9.4308) (2.9042, 9.4136) (3.007, 9.4019) knots 0 0 0 0 1 1 1 1
  spline S67 degree 3 poles (3.2397, 9.3707) (3.2949, 9.3587) (3.3002, 9.298) (3.2504, 9.2482) knots 0 0 0 0 1 1 1 1
  spline S68 degree 3 poles (4.5002, 10.0683) (4.1645, 10.4099) (3.5131, 10.851) (2.7089, 11.2812) knots 0 0 0 0 1 1 1 1
  spline S69 degree 3 poles (4.6393, 11.6781) (4.6263, 11.6781) (4.5381, 11.7622) (4.4433, 11.8651) knots 0 0 0 0 1 1 1 1
  spline S70 degree 3 poles (2.9891, 12.1417) (3.0301, 12.0832) (3.0303, 12.0257) (2.9896, 12.0101) knots 0 0 0 0 1 1 1 1
  line L26 (4.4433, 11.8651) -> (4.271, 12.0522)
  spline S71 degree 3 poles (1.8961, 11.8203) (1.7913, 11.8203) (1.6777, 11.8147) (1.6436, 11.8079) knots 0 0 0 0 1 1 1 1
  spline S72 degree 3 poles (1.9646, 10.5876) (1.9646, 10.574) (1.9264, 10.5553) (1.8796, 10.546) knots 0 0 0 0 1 1 1 1
  line L27 (1.8796, 10.546) -> (1.7946, 10.5292)
  spline S73 degree 3 poles (2.7089, 11.2812) (2.5424, 11.3703) (2.4958, 11.4037) (2.5195, 11.417) knots 0 0 0 0 1 1 1 1
  spline S74 degree 3 poles (1.6579, 10.9309) (1.6686, 10.9116) (1.7419, 10.832) (1.821, 10.754) knots 0 0 0 0 1 1 1 1
  spline S75 degree 3 poles (3.8239, 9.279) (4.1927, 9.3756) (4.4295, 9.5421) (4.5552, 9.7934) knots 0 0 0 0 1 1 1 1
  line L28 (4.5552, 9.7934) -> (4.6278, 9.9384)
  spline S76 degree 3 poles (4.0645, 11.9698) (3.9187, 12.1168) (3.8747, 12.1432) (3.8747, 12.0838) knots 0 0 0 0 1 1 1 1
  spline S77 degree 3 poles (3.4213, 12.0266) (3.4013, 12.0101) (3.3542, 12.0242) (3.2334, 12.0831) knots 0 0 0 0 1 1 1 1
  spline S78 degree 3 poles (3.8006, 11.9625) (3.783, 11.9625) (3.7128, 12.0044) (3.6447, 12.0556) knots 0 0 0 0 1 1 1 1
  spline S79 degree 3 poles (1.7614, 11.4022) (1.7614, 11.3837) (1.725, 11.3734) (1.6446, 11.3692) knots 0 0 0 0 1 1 1 1
  spline S80 degree 3 poles (1.6949, 10.9548) (1.6461, 10.9645) (1.6411, 10.9613) (1.6579, 10.9309) knots 0 0 0 0 1 1 1 1
  line L29 (4.6278, 9.9384) -> (4.5002, 10.0683)
  spline S81 degree 3 poles (3.6447, 12.0556) (3.5159, 12.1525) (3.3756, 12.2338) (3.4226, 12.1843) knots 0 0 0 0 1 1 1 1
  spline S82 degree 3 poles (3.0145, 12.1747) (2.9581, 12.1874) (2.9576, 12.1867) (2.9891, 12.1417) knots 0 0 0 0 1 1 1 1
  spline S83 degree 3 poles (2.9896, 12.0101) (2.9722, 12.0034) (2.8922, 12.0166) (2.8118, 12.0395) knots 0 0 0 0 1 1 1 1
  spline S84 degree 3 poles (2.0129, 11.9769) (2.0049, 11.9689) (2.0182, 11.9413) (2.0425, 11.9154) knots 0 0 0 0 1 1 1 1
  spline S85 degree 3 poles (2.112, 10.2869) (2.1968, 10.2324) (2.185, 10.1823) (2.0836, 10.1661) knots 0 0 0 0 1 1 1 1
  line L30 (2.3461, 9.7546) -> (2.445, 9.713)
  spline S86 degree 3 poles (4.6921, 11.7513) (4.676, 11.711) (4.6522, 11.6781) (4.6393, 11.6781) knots 0 0 0 0 1 1 1 1
  line L31 (1.9993, 10.1526) -> (2.0671, 10.1026)
  spline S87 degree 3 poles (3.007, 9.4019) (3.1099, 9.3902) (3.2146, 9.3762) (3.2397, 9.3707) knots 0 0 0 0 1 1 1 1
  line L32 (1.6446, 11.3692) -> (1.5278, 11.3631)
  spline S88 degree 3 poles (4.8839, 10.2242) (4.9661, 10.2448) (5.1446, 10.4393) (5.1818, 10.5488) knots 0 0 0 0 1 1 1 1
  spline S89 degree 3 poles (3.9148, 9.253) (3.6892, 9.1879) (3.2701, 9.1432) (3.1584, 9.1724) knots 0 0 0 0 1 1 1 1
  line L33 (4.7213, 11.8245) -> (4.6921, 11.7513)
  spline S90 degree 3 poles (2.5946, 11.974) (2.5946, 11.9111) (2.5628, 11.908) (2.3875, 11.9534) knots 0 0 0 0 1 1 1 1
  spline S91 degree 3 poles (2.4876, 9.8426) (2.4833, 9.8295) (2.4498, 9.8043) (2.413, 9.7867) knots 0 0 0 0 1 1 1 1
  spline S92 degree 3 poles (2.6809, 9.6266) (2.8293, 9.5781) (2.861, 9.5282) (2.7731, 9.4812) knots 0 0 0 0 1 1 1 1
  spline S93 degree 3 poles (2.0425, 11.9154) (2.1205, 11.8323) (2.1021, 11.8203) (1.8961, 11.8203) knots 0 0 0 0 1 1 1 1
  spline S94 degree 3 poles (3.2334, 12.0831) (3.1447, 12.1264) (3.0462, 12.1676) (3.0145, 12.1747) knots 0 0 0 0 1 1 1 1
  spline S95 degree 3 poles (5.1818, 10.5488) (5.2844, 10.8506) (5.1495, 11.2864) (4.8289, 11.6893) knots 0 0 0 0 1 1 1 1
  spline S96 degree 3 poles (2.3875, 11.9534) (2.2575, 11.9871) (2.0369, 12.0009) (2.0129, 11.9769) knots 0 0 0 0 1 1 1 1
  spline S97 degree 3 poles (3.8747, 12.0838) (3.8747, 12.0227) (3.838, 11.9625) (3.8006, 11.9625) knots 0 0 0 0 1 1 1 1
  spline S98 degree 3 poles (1.6954, 11.1955) (1.7876, 11.1034) (1.863, 11.0186) (1.863, 11.0071) knots 0 0 0 0 1 1 1 1
  spline S99 degree 3 poles (2.5732, 12.0661) (2.5849, 12.0442) (2.5946, 12.0027) (2.5946, 11.974) knots 0 0 0 0 1 1 1 1
  spline S100 degree 3 poles (2.8118, 12.0395) (2.5602, 12.1111) (2.5484, 12.1124) (2.5732, 12.0661) knots 0 0 0 0 1 1 1 1
  spline S101 degree 3 poles (2.5195, 11.417) (2.5403, 11.4286) (2.6149, 11.4114) (2.7404, 11.3659) knots 0 0 0 0 1 1 1 1
  line L34 (1.5817, 11.7955) -> (1.6409, 11.6994)
  spline S102 degree 3 poles (1.6409, 11.6994) (1.7004, 11.6026) (1.7614, 11.4522) (1.7614, 11.4022) knots 0 0 0 0 1 1 1 1
  spline S103 degree 3 poles (1.9254, 10.426) (1.9973, 10.3693) (2.0812, 10.3066) (2.112, 10.2869) knots 0 0 0 0 1 1 1 1
  line L35 (4.271, 12.0522) -> (4.2608, 11.9739)
  spline S104 degree 3 poles (2.6474, 12.501) (2.718, 12.5479) (2.9479, 12.5672) (3.0427, 12.5342) knots 0 0 0 0 1 1 1 1
  spline S105 degree 3 poles (3.77, 12.5062) (3.8886, 12.5147) (3.921, 12.509) (4.0104, 12.4637) knots 0 0 0 0 1 1 1 1
  spline S106 degree 3 poles (1.7109, 12.236) (1.8205, 12.3197) (1.9129, 12.3484) (2.0732, 12.3485) knots 0 0 0 0 1 1 1 1
  spline S107 degree 3 poles (6.823, 12.4218) (6.8805, 12.4126) (6.9191, 12.4218) (6.9902, 12.4615) knots 0 0 0 0 1 1 1 1
  spline S108 degree 3 poles (7.4758, 12.5392) (7.5704, 12.5805) (7.7594, 12.5818) (7.837, 12.5417) knots 0 0 0 0 1 1 1 1
  spline S109 degree 3 poles (3.4384, 9.2248) (3.561, 9.2312) (3.7345, 9.2556) (3.8239, 9.279) knots 0 0 0 0 1 1 1 1
  spline S110 degree 3 poles (8.7681, 12.3834) (8.7898, 12.3644) (8.8619, 12.35) (8.9649, 12.3442) knots 0 0 0 0 1 1 1 1
  spline S111 degree 3 poles (1.2336, 12.0196) (1.2832, 12.101) (1.4139, 12.1647) (1.5327, 12.1653) knots 0 0 0 0 1 1 1 1
  spline S112 degree 3 poles (1.5327, 12.1653) (1.5993, 12.1656) (1.6398, 12.1817) (1.7109, 12.236) knots 0 0 0 0 1 1 1 1
  spline S113 degree 3 poles (4.1829, 12.4226) (4.2955, 12.4408) (4.4186, 12.3954) (4.5244, 12.2964) knots 0 0 0 0 1 1 1 1
  spline S114 degree 3 poles (6.298, 12.2064) (6.367, 12.2064) (6.3953, 12.2207) (6.4763, 12.2964) knots 0 0 0 0 1 1 1 1
  line L36 (1.6954, 11.0133) -> (1.8122, 11.0056)
  spline S115 degree 3 poles (8.4967, 12.4696) (8.5897, 12.4686) (8.7172, 12.4281) (8.7681, 12.3834) knots 0 0 0 0 1 1 1 1
  spline S116 degree 3 poles (3.2504, 9.2482) (3.2173, 9.215) (3.2273, 9.2138) (3.4384, 9.2248) knots 0 0 0 0 1 1 1 1
  spline S117 degree 3 poles (1.924, 9.736) (1.924, 9.7528) (1.9049, 9.7768) (1.8816, 9.7893) knots 0 0 0 0 1 1 1 1
  spline S118 degree 3 poles (8.9649, 12.3442) (9.1359, 12.3346) (9.2549, 12.2902) (9.3287, 12.2085) knots 0 0 0 0 1 1 1 1
  spline S119 degree 3 poles (9.3287, 12.2085) (9.3572, 12.177) (9.392, 12.1656) (9.4608, 12.1653) knots 0 0 0 0 1 1 1 1
  spline S120 degree 3 poles (7.2414, 12.5097) (7.35, 12.5073) (7.4241, 12.5166) (7.4758, 12.5392) knots 0 0 0 0 1 1 1 1
  spline S121 degree 3 poles (1.2034, 11.2295) (1.1413, 11.352) (1.138, 11.4494) (1.1924, 11.5559) knots 0 0 0 0 1 1 1 1
  spline S122 degree 3 poles (2.8679, 12.076) (2.9233, 12.0591) (2.973, 12.0497) (2.9783, 12.055) knots 0 0 0 0 1 1 1 1
  spline S123 degree 3 poles (1.5583, 11.7389) (1.4768, 11.8534) (1.4903, 11.8609) (1.7754, 11.8609) knots 0 0 0 0 1 1 1 1
  spline S124 degree 3 poles (2.6163, 9.1073) (2.5097, 9.1307) (2.3825, 9.2279) (2.3425, 9.3165) knots 0 0 0 0 1 1 1 1
  spline S125 degree 3 poles (2.3425, 9.3165) (2.3152, 9.3772) (2.2894, 9.4035) (2.2487, 9.4125) knots 0 0 0 0 1 1 1 1
  spline S126 degree 3 poles (2.2435, 12.3892) (2.3072, 12.4393) (2.4349, 12.4752) (2.5226, 12.4676) knots 0 0 0 0 1 1 1 1
  spline S127 degree 3 poles (1.242, 11.0588) (1.2517, 11.1106) (1.2422, 11.1531) (1.2034, 11.2295) knots 0 0 0 0 1 1 1 1
  spline S128 degree 3 poles (7.837, 12.5417) (7.8808, 12.5191) (7.9094, 12.5165) (7.9491, 12.5316) knots 0 0 0 0 1 1 1 1
  spline S129 degree 3 poles (9.4608, 12.1653) (9.5861, 12.1647) (9.7163, 12.1027) (9.767, 12.0196) knots 0 0 0 0 1 1 1 1
  spline S130 degree 3 poles (1.3957, 10.5815) (1.3957, 10.6398) (1.3782, 10.6904) (1.3377, 10.7498) knots 0 0 0 0 1 1 1 1
  line L37 (1.8122, 11.0056) -> (1.698, 11.1132)
  spline S131 degree 3 poles (2.0596, 12.0367) (2.1496, 12.0473) (2.4249, 12.0077) (2.5233, 11.9699) knots 0 0 0 0 1 1 1 1
  spline S132 degree 3 poles (9.8094, 11.5639) (9.8634, 11.4579) (9.8596, 11.3387) (9.7985, 11.2238) knots 0 0 0 0 1 1 1 1
  spline S133 degree 3 poles (2.5233, 11.9699) (2.5708, 11.9517) (2.5598, 12.005) (2.504, 12.0632) knots 0 0 0 0 1 1 1 1
  spline S134 degree 3 poles (1.5989, 10.1696) (1.5989, 10.2095) (1.5762, 10.249) (1.5253, 10.2974) knots 0 0 0 0 1 1 1 1
  spline S135 degree 3 poles (1.1924, 11.5559) (1.2241, 11.6181) (1.2285, 11.6469) (1.2127, 11.6885) knots 0 0 0 0 1 1 1 1
  spline S136 degree 3 poles (1.9747, 11.922) (1.9029, 11.997) (1.92, 12.0201) (2.0596, 12.0367) knots 0 0 0 0 1 1 1 1
  spline S137 degree 3 poles (1.2127, 11.6885) (1.178, 11.7797) (1.1885, 11.9456) (1.2336, 12.0196) knots 0 0 0 0 1 1 1 1
  spline S138 degree 3 poles (2.4699, 12.141) (2.4869, 12.1685) (2.6546, 12.1411) (2.8679, 12.076) knots 0 0 0 0 1 1 1 1
  spline S139 degree 3 poles (2.9783, 12.055) (2.9836, 12.0604) (2.9589, 12.0948) (2.9234, 12.1315) knots 0 0 0 0 1 1 1 1
  spline S140 degree 3 poles (2.4965, 8.9757) (2.6673, 9.0899) (2.672, 9.095) (2.6163, 9.1073) knots 0 0 0 0 1 1 1 1
  spline S141 degree 3 poles (1.5253, 10.2974) (1.436, 10.3825) (1.3957, 10.4708) (1.3957, 10.5815) knots 0 0 0 0 1 1 1 1
  spline S142 degree 3 poles (3.5484, 12.5343) (3.6136, 12.5051) (3.6643, 12.4987) (3.77, 12.5062) knots 0 0 0 0 1 1 1 1
  spline S143 degree 3 poles (4.0104, 12.4637) (4.0856, 12.4256) (4.1325, 12.4144) (4.1829, 12.4226) knots 0 0 0 0 1 1 1 1
  spline S144 degree 3 poles (4.7026, 12.2064) (4.8097, 12.2064) (4.9861, 12.0791) (5.1448, 11.8873) knots 0 0 0 0 1 1 1 1
  spline S145 degree 3 poles (5.1448, 11.8873) (5.2515, 11.7583) (5.48, 11.3445) (5.48, 11.2802) knots 0 0 0 0 1 1 1 1
  spline S146 degree 3 poles (5.566, 11.3887) (5.7365, 11.8095) (6.0918, 12.2064) (6.298, 12.2064) knots 0 0 0 0 1 1 1 1
  line L38 (2.7731, 9.4812) -> (2.7281, 9.4571)
  spline S147 degree 3 poles (3.0923, 12.1969) (3.1744, 12.1693) (3.272, 12.1282) (3.3092, 12.1055) knots 0 0 0 0 1 1 1 1
  spline S148 degree 3 poles (1.8816, 9.7893) (1.74, 9.865) (1.5989, 10.0549) (1.5989, 10.1696) knots 0 0 0 0 1 1 1 1
  spline S149 degree 3 poles (2.5226, 12.4676) (2.562, 12.4642) (2.6122, 12.4777) (2.6474, 12.501) knots 0 0 0 0 1 1 1 1
  spline S150 degree 3 poles (5.48, 11.2802) (5.48, 11.2167) (5.5133, 11.2588) (5.566, 11.3887) knots 0 0 0 0 1 1 1 1
  spline S151 degree 3 poles (6.4763, 12.2964) (6.5836, 12.3968) (6.7049, 12.4407) (6.823, 12.4218) knots 0 0 0 0 1 1 1 1
  spline S152 degree 3 poles (2.2487, 9.4125) (2.102, 9.4447) (1.924, 9.622) (1.924, 9.736) knots 0 0 0 0 1 1 1 1
  spline S153 degree 3 poles (2.504, 12.0632) (2.4733, 12.0953) (2.4602, 12.1252) (2.4699, 12.141) knots 0 0 0 0 1 1 1 1
  line L39 (2.7281, 9.4571) -> (2.7741, 9.4401)
  spline S154 degree 3 poles (4.5244, 12.2964) (4.6053, 12.2207) (4.6336, 12.2064) (4.7026, 12.2064) knots 0 0 0 0 1 1 1 1
  spline S155 degree 3 poles (8.335, 12.5112) (8.3788, 12.4888) (8.4516, 12.4701) (8.4967, 12.4696) knots 0 0 0 0 1 1 1 1
  spline S156 degree 3 poles (7.9491, 12.5316) (8.0419, 12.5668) (8.247, 12.556) (8.335, 12.5112) knots 0 0 0 0 1 1 1 1
  spline S157 degree 3 poles (2.0732, 12.3485) (2.1609, 12.3486) (2.2054, 12.3592) (2.2435, 12.3892) knots 0 0 0 0 1 1 1 1
  spline S158 degree 3 poles (2.9234, 12.1315) (2.8008, 12.2579) (2.8518, 12.2776) (3.0923, 12.1969) knots 0 0 0 0 1 1 1 1
  spline S159 degree 3 poles (3.0427, 12.5342) (3.0925, 12.5168) (3.1187, 12.5185) (3.1643, 12.5421) knots 0 0 0 0 1 1 1 1
  spline S160 degree 3 poles (1.9194, 8.3954) (2.0271, 8.5728) (2.2911, 8.8383) (2.4965, 8.9757) knots 0 0 0 0 1 1 1 1
  spline S161 degree 3 poles (6.9902, 12.4615) (7.0695, 12.5058) (7.1052, 12.5127) (7.2414, 12.5097) knots 0 0 0 0 1 1 1 1
  spline S162 degree 3 poles (1.3377, 10.7498) (1.2608, 10.8624) (1.2262, 10.9742) (1.242, 11.0588) knots 0 0 0 0 1 1 1 1
  spline S163 degree 3 poles (3.1643, 12.5421) (3.2463, 12.5845) (3.4454, 12.5804) (3.5484, 12.5343) knots 0 0 0 0 1 1 1 1
  spline S164 degree 3 poles (2.1195, 7.9187) (2.199, 8.1564) (2.2998, 8.3185) (2.481, 8.5) knots 0 0 0 0 1 1 1 1
  spline S165 degree 3 poles (2.8384, 8.759) (3.1037, 8.8887) (3.2251, 8.9172) (3.5598, 8.9285) knots 0 0 0 0 1 1 1 1
  spline S166 degree 3 poles (8.8344, 7.2219) (8.8062, 7.1479) (8.7189, 7.1488) (8.5585, 7.2249) knots 0 0 0 0 1 1 1 1
  spline S167 degree 3 poles (3.0111, 7.7326) (2.4277, 7.2683) (2.1091, 7.1117) (2.0429, 7.257) knots 0 0 0 0 1 1 1 1
  spline S168 degree 3 poles (2.2619, 7.281) (2.6819, 7.4556) (3.7895, 8.4235) (3.9654, 8.7696) knots 0 0 0 0 1 1 1 1
  spline S169 degree 3 poles (9.6922, 4.1089) (9.7305, 4.2593) (9.7575, 4.317) (9.8442, 4.434) knots 0 0 0 0 1 1 1 1
  spline S170 degree 3 poles (3.1545, 8.8373) (2.5306, 8.6567) (2.1559, 8.1956) (2.0867, 7.5233) knots 0 0 0 0 1 1 1 1
  spline S171 degree 3 poles (9.9898, 6.5065) (10.0961, 6.3207) (10.1618, 6.1614) (10.2182, 5.9527) knots 0 0 0 0 1 1 1 1
  spline S172 degree 3 poles (9.6753, 10.7626) (9.6206, 10.6812) (9.605, 10.6374) (9.605, 10.5653) knots 0 0 0 0 1 1 1 1
  spline S173 degree 3 poles (9.6236, 3.7012) (9.5773, 3.5678) (9.5233, 3.3809) (9.5035, 3.2859) knots 0 0 0 0 1 1 1 1
  spline S174 degree 3 poles (5.5511, 0.4299) (5.3947, 0.4269) (5.2392, 0.4288) (5.2057, 0.4341) knots 0 0 0 0 1 1 1 1
  spline S175 degree 3 poles (7.109, 1.1854) (7.4209, 1.3113) (7.7213, 1.4803) (8.0403, 1.7091) knots 0 0 0 0 1 1 1 1
  spline S176 degree 3 poles (7.705, 8.8552) (8.2311, 8.7191) (8.6146, 8.3577) (8.7693, 7.8524) knots 0 0 0 0 1 1 1 1
  spline S177 degree 3 poles (6.0083, 0.4804) (5.8779, 0.4463) (5.766, 0.434) (5.5511, 0.4299) knots 0 0 0 0 1 1 1 1
  line L40 (8.3402, 9.0836) -> (8.4392, 9.0226)
  spline S178 degree 3 poles (8.3169, 1.8754) (8.4816, 1.9424) (8.7072, 2.1028) (8.8854, 2.2796) knots 0 0 0 0 1 1 1 1
  spline S179 degree 3 poles (8.7693, 7.8524) (8.824, 7.6739) (8.8628, 7.2968) (8.8344, 7.2219) knots 0 0 0 0 1 1 1 1
  spline S180 degree 3 poles (3.5598, 8.9285) (4.0246, 8.9441) (4.0886, 8.9123) (3.9871, 8.7162) knots 0 0 0 0 1 1 1 1
  spline S181 degree 3 poles (9.0721, 9.6998) (9.038, 9.586) (8.9253, 9.4756) (8.7971, 9.4303) knots 0 0 0 0 1 1 1 1
  spline S182 degree 3 poles (3.9871, 8.7162) (3.9091, 8.5654) (3.3519, 8.0039) (3.0111, 7.7326) knots 0 0 0 0 1 1 1 1
  spline S183 degree 3 poles (8.9456, 2.2578) (8.746, 2.0573) (8.5796, 1.9357) (8.3714, 1.8383) knots 0 0 0 0 1 1 1 1
  spline S184 degree 3 poles (8.3714, 1.8383) (8.2981, 1.8039) (8.1365, 1.7045) (8.0122, 1.6173) knots 0 0 0 0 1 1 1 1
  spline S185 degree 3 poles (7.5375, 8.0447) (8.084, 7.5559) (8.6062, 7.195) (8.7414, 7.2125) knots 0 0 0 0 1 1 1 1
  spline S186 degree 3 poles (8.6776, 9.3517) (8.6501, 9.2629) (8.5773, 9.1912) (8.4612, 9.1385) knots 0 0 0 0 1 1 1 1
  spline S187 degree 3 poles (8.6269, 8.0792) (8.562, 8.2133) (8.509, 8.2854) (8.3787, 8.4165) knots 0 0 0 0 1 1 1 1
  spline S188 degree 3 poles (9.5035, 3.2859) (9.4209, 2.8889) (9.2376, 2.5511) (8.9456, 2.2578) knots 0 0 0 0 1 1 1 1
  spline S189 degree 3 poles (9.4656, 10.2775) (9.4434, 10.2656) (9.4192, 10.2139) (9.404, 10.1458) knots 0 0 0 0 1 1 1 1
  spline S190 degree 3 poles (9.7603, 11.0691) (9.7791, 10.9749) (9.7518, 10.8761) (9.6753, 10.7626) knots 0 0 0 0 1 1 1 1
  spline S191 degree 3 poles (8.7971, 9.4303) (8.7283, 9.406) (8.6857, 9.378) (8.6776, 9.3517) knots 0 0 0 0 1 1 1 1
  spline S192 degree 3 poles (6.0251, 0.5408) (6.3327, 0.6308) (6.6165, 0.7931) (6.8531, 1.0145) knots 0 0 0 0 1 1 1 1
  spline S193 degree 3 poles (6.8482, 8.842) (6.8765, 8.9157) (7.4378, 8.9244) (7.705, 8.8552) knots 0 0 0 0 1 1 1 1
  spline S194 degree 3 poles (9.7985, 11.2238) (9.7631, 11.1571) (9.7518, 11.1115) (9.7603, 11.0691) knots 0 0 0 0 1 1 1 1
  spline S195 degree 3 poles (9.767, 12.0196) (9.8115, 11.9466) (9.8227, 11.78) (9.7891, 11.6914) knots 0 0 0 0 1 1 1 1
  spline S196 degree 3 poles (8.4392, 9.0226) (9.0103, 8.6707) (9.3189, 8.1447) (9.3549, 7.4617) knots 0 0 0 0 1 1 1 1
  spline S197 degree 3 poles (6.9157, 0.9846) (6.6287, 0.7311) (6.3277, 0.5639) (6.0083, 0.4804) knots 0 0 0 0 1 1 1 1
  spline S198 degree 3 poles (8.8854, 2.2796) (9.188, 2.5797) (9.3687, 2.9119) (9.4532, 3.3234) knots 0 0 0 0 1 1 1 1
  spline S199 degree 3 poles (6.8531, 1.0145) (6.9382, 1.0941) (7.0229, 1.1506) (7.109, 1.1854) knots 0 0 0 0 1 1 1 1
  spline S200 degree 3 poles (9.8929, 4.3977) (9.8105, 4.289) (9.7798, 4.2263) (9.748, 4.1018) knots 0 0 0 0 1 1 1 1
  line L41 (8.4612, 9.1385) -> (8.3402, 9.0836)